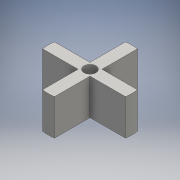
# Autodesk Inventor part: Single Spoke
Saved by Autodesk Inventor 2016 (Build 200138000, 138)
## iProperties
Created: 2016-12-01
Part Number: Single Spoke
Material: Generic
Document SubType Name: Modeling
Designer: Kevin
Density: 1 g/cm^3
Appearance: Default
Author: Kevin
Autodesk Inventor part; units mm, degrees
ref_plane "YZ Plane" through (0, 0, 0) normal (1, 0, 0) x (0, 1, 0)
ref_plane "XZ Plane" through (0, 0, 0) normal (0, 1, 0) x (-1, 0, 0)
ref_plane "XY Plane" through (0, 0, 0) normal (0, 0, 1) x (1, 0, 0)
sketch "Sketch1" plane through (0, 0, 0) normal (0, 0, 1) x (1, 0, 0)
  circle A0 centre (0, 0) radius 44.45
  circle A1 centre (0, 0) radius 6.35
  line L0 (-43.9941, 6.35) -> (-6.35, 6.35)
  line L1 (-43.9941, -6.35) -> (-6.35, -6.35)
  line L2 (6.35, -6.35) -> (43.9941, -6.35)
  line L3 (6.35, 6.35) -> (43.9941, 6.35)
  line L4 (-6.35, 6.35) -> (-6.35, 43.9941)
  line L5 (6.35, 6.35) -> (6.35, 43.9941)
  line L6 (6.35, -6.35) -> (6.35, -43.9941)
  line L7 (-6.35, -6.35) -> (-6.35, -43.9941)
  circle A2 centre (0, 0) radius 8.9803
  dimension "d0" = 88.9
  dimension "d1" = 12.7
  constraints: 16 end point, 5 point on line, 2 coincident, 1 centre point, 1 parallel, 1 vertical, 13 other
  measures "d1" diameter of A1
extrude "Extrusion2" add sketch "Sketch1" along normal blind 38.1 contours A0 L2 A2 L3 | L5 A2 L4 A0 | A2 | A0 L7 A2 L6 | A2 L1 A0 L0
body "Solid2"
